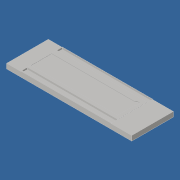
# Autodesk Inventor part: Button Fixture Base
Saved by Autodesk Inventor 2016 (Build 200138000, 138)
## iProperties
Created: 2016-07-07
Part Number: Button Fixture Base
Material: Generic
Document SubType Name: Modeling
Designer: Sam Clay
Density: 1 g/cm^3
Appearance: Default
Author: Sam Clay
Autodesk Inventor part; units mm, degrees
ref_plane "YZ Plane" through (0, 0, 0) normal (1, 0, 0) x (0, 1, 0)
ref_plane "XZ Plane" through (0, 0, 0) normal (0, 1, 0) x (-1, 0, 0)
ref_plane "XY Plane" through (0, 0, 0) normal (0, 0, 1) x (1, 0, 0)
sketch "Sketch1" plane through (0, 0, 0) normal (0, 1, 0) x (-1, 0, 0)
  line L0 (0, 0) -> (330.2, 0)
  line L1 (330.2, 0) -> (330.2, 152.4)
  line L2 (330.2, 152.4) -> (0, 152.4)
  line L3 (0, 152.4) -> (0, 0)
  line L4 (330.2, 0) -> (381, 0)
  line L5 (381, 0) -> (381, 152.4)
  line L6 (381, 152.4) -> (330.2, 152.4)
  line L7 (330.2, 152.4) -> (330.2, 0)
  line L8 (0, 0) -> (-76.2, 0)
  line L9 (-76.2, 0) -> (-76.2, 152.4)
  line L10 (-76.2, 152.4) -> (0, 152.4)
  line L11 (0, 152.4) -> (0, 0)
  dimension "d0" = 330.2
  dimension "d1" = 152.4
  dimension "d2" = 50.8
  dimension "d3" = 76.2
  constraints: 24 end point, 6 parallel, 3 horizontal, 3 perpendicular, 2 point on line
  measures "d0" distance of L2.end L1.end
  measures "d1" distance of L1.end L0.end
  measures "d2" distance of L6.end L5.end
  measures "d3" distance of L9.end L10.end
extrude "Extrusion1" add sketch "Sketch1" along normal blind 19.05 contours L3 L2 L1 L0
extrude "Extrusion2" add sketch "Sketch1" along normal blind 17.78 contours L8 L9 L10 L3 | L1 L6 L5 L4
sketch "Sketch2" plane through (0, 19.05, 0) normal (0, 1, 0) x (1, 0, 0)
  line L0 (-330.2, 0) -> (-330.2, -152.4) projected
  line L1 (0, 0) -> (-330.2, 0)
  line L2 (-330.2, 0) -> (-330.2, -0.254)
  line L3 (-330.2, -0.254) -> (0, -0.254)
  line L4 (0, -0.254) -> (0, 0)
  line L5 (0, -0.254) -> (-330.2, -0.254)
  line L6 (-330.2, -0.254) -> (-330.2, -20.066)
  line L7 (-330.2, -20.066) -> (0, -20.066)
  line L8 (0, -20.066) -> (0, -0.254)
  line L9 (0, -20.066) -> (-330.2, -20.066)
  line L10 (-330.2, -20.066) -> (-330.2, -39.116)
  line L11 (-330.2, -39.116) -> (0, -39.116)
  line L12 (0, -39.116) -> (0, -20.066)
  line L13 (0, -39.116) -> (-330.2, -39.116)
  line L14 (-330.2, -39.116) -> (-330.2, -115.316)
  line L15 (-330.2, -115.316) -> (0, -115.316)
  line L16 (0, -115.316) -> (0, -39.116)
  line L17 (0, -115.316) -> (-330.2, -115.316)
  line L18 (-330.2, -115.316) -> (-330.2, -128.016)
  line L19 (-330.2, -128.016) -> (0, -128.016)
  line L20 (0, -128.016) -> (0, -115.316)
  line L21 (0, -128.016) -> (-330.2, -128.016)
  line L22 (-330.2, -128.016) -> (-330.2, -147.828)
  line L23 (-330.2, -147.828) -> (0, -147.828)
  line L24 (0, -147.828) -> (0, -128.016)
  line L25 (0, -147.828) -> (-330.2, -147.828)
  line L26 (-330.2, -147.828) -> (-330.2, -151.003)
  line L27 (-330.2, -151.003) -> (0, -151.003)
  line L28 (0, -151.003) -> (0, -147.828)
  line L29 (0, -152.4) -> (0, 0) projected
  line L30 (0, 0) -> (-12.7, 0)
  line L31 (-12.7, 0) -> (-12.7, -115.316)
  line L32 (-12.7, -115.316) -> (0, -115.316)
  line L33 (0, -115.316) -> (0, 0)
  circle A0 centre (-16.2783, -42.291) radius 8.89
  point P0 (-12.7, -39.116)
  dimension "d8" = 0.254
  dimension "d9" = 19.812
  dimension "d10" = 19.05
  dimension "d11" = 76.2
  dimension "d12" = 12.7
  dimension "d13" = 19.812
  dimension "d14" = 3.175
  dimension "d15" = 12.7
  dimension "d16" = 17.78
  dimension "d21" = 3.175
  constraints: 64 end point, 16 parallel, 10 point on line, 8 horizontal, 8 perpendicular, 1 centre point
  measures "d8" distance of L2.end L1.end
  measures "d9" distance of L6.end L5.end
  measures "d10" distance of L10.end L9.end
  measures "d11" distance of L14.end L13.end
  measures "d12" distance of L18.end L17.end
  measures "d13" distance of L22.end L21.end
  measures "d14" distance of L26.end L25.end
  measures "d15" distance of L32.end L31.end
  measures "d16" diameter of A0
  measures "d21" distance from line of L13 A0.centre
extrude "Extrusion3" cut sketch "Sketch2" against normal blind 7.62 contours L3 L31 L7 L0 | L3 L8 L7 L31 | L19 L24 L23 L0
extrude "Extrusion4" cut sketch "Sketch2" against normal blind 3.175 contours L11 A0 L31 L15 L0 | A0 L31 L11 | L11 L31 A0 | A0 L11 L31 | L11 A0 L31
body "Solid1"
